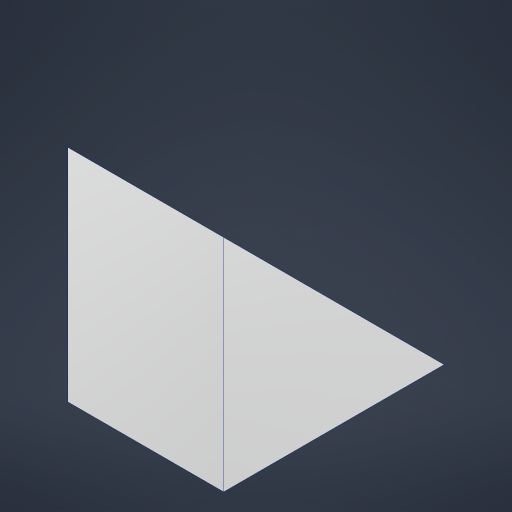
# Autodesk Inventor part: STRU_011_BilletWedge
Saved by Autodesk Inventor 2024.2 (Build 282272000, 272)
## iProperties
Created: 2024-07-25
Part Number: STRU_011_BilletWedge
Material: Aluminum 6061
Document SubType Name: Modeling
Designer: Bryan
Density: 2.7 g/cm^3
Appearance: Aluminum - Flat
Author: Bryan
Autodesk Inventor part; units mm, degrees
ref_plane "YZ Plane" through (0, 0, 0) normal (1, 0, 0) x (0, 1, 0)
ref_plane "XZ Plane" through (0, 0, 0) normal (0, 1, 0) x (-1, 0, 0)
ref_plane "XY Plane" through (0, 0, 0) normal (0, 0, 1) x (1, 0, 0)
sketch "Sketch1" plane through (0, 0, 0) normal (0, 1, 0) x (-1, 0, 0)
  line L0 (-9.525, -13.4747) -> (9.525, -13.4747)
  line L1 (9.525, -13.4747) -> (9.525, 13.4747)
  line L2 (9.525, 13.4747) -> (-9.525, 13.4747)
  line L3 (-9.525, 13.4747) -> (-9.525, -13.4747)
  line L4 (-9.525, -13.4747) -> (9.525, 13.4747) construction
  line L5 (9.525, -13.4747) -> (-9.525, 13.4747) construction
  point P0 (0, 0)
  dimension "d0" = 19.05
  dimension "d1" = 26.9494
  constraints: 12 end point, 2 midpoint, 2 parallel, 1 horizontal, 1 perpendicular
  measures "d0" distance of L2.end L1.end
  measures "d1" distance of L1.end L0.end
extrude "Extrusion1" add sketch "Sketch1" along normal blind 26.9494
sketch "Sketch2" plane through (9.525, 0, 13.4747) normal (1, 0, 0) x (0, 0, -1)
  line L0 (26.9494, 26.9494) -> (0, 26.9494) projected
  line L1 (0, 26.9494) -> (26.9494, 0)
  line L2 (0, 0) -> (26.9494, 0) projected
  line L3 (26.9494, 0) -> (26.9494, 26.9494) projected
  line L4 (0, 26.9494) -> (26.9494, 26.9494) projected
  line L5 (0, 0) -> (0, 26.9494) projected
  point P0 (13.4747, 0)
  constraints: 2 end point
extrude "Extrusion2" cut sketch "Sketch2" against normal blind 19.05 contours L3 L1 L0
sketch "Sketch3" plane through (0, 0, 0) normal (0, -1, 0) x (1, 0, 0)
  circle A0 centre (0, 0) radius 2.0193
  dimension "d6" = 4.0386
  constraints: 1 centre point, 1 coincident
  measures "d6" diameter of A0
extrude "Extrusion3" cut sketch "Sketch3" against normal blind 19.05
thread "Thread1" size "10-32 UNF" class "2B" standard "ANSI Unified Screw Threads" full length
body "Solid1"
